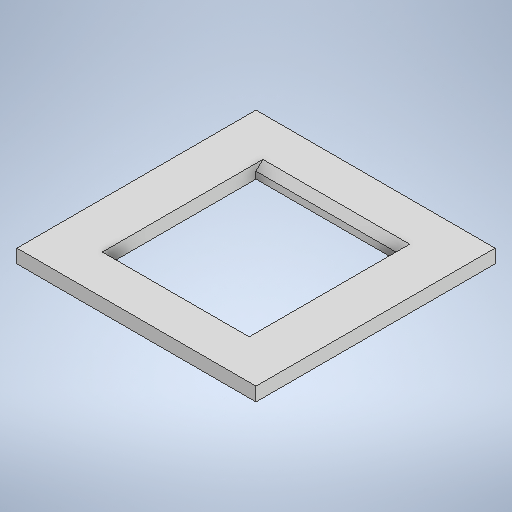
# Autodesk Inventor part: Plug_tester
Saved by Autodesk Inventor 2025 (Build 290162000, 162)
## iProperties
Created: 2024-12-15
Part Number: Plug_tester
Material: Generic
Document SubType Name: Modeling
Designer: ethan
Density: 1 g/cm^3
Appearance: Default
Author: ethan
Autodesk Inventor part; units mm, degrees
ref_plane "YZ Plane" through (0, 0, 0) normal (1, 0, 0) x (0, 1, 0)
ref_plane "XZ Plane" through (0, 0, 0) normal (0, 1, 0) x (-1, 0, 0)
ref_plane "XY Plane" through (0, 0, 0) normal (0, 0, 1) x (1, 0, 0)
sketch "Sketch1" plane through (0, 0, 0) normal (0, 1, 0) x (-1, 0, 0)
  line L0 (0, 0) -> (35, 0)
  line L1 (35, 0) -> (35, -35)
  line L2 (35, -35) -> (0, -35)
  line L3 (0, -35) -> (0, 0)
  line L4 (6.75, -6.75) -> (28.25, -6.75)
  line L5 (28.25, -6.75) -> (28.25, -28.25)
  line L6 (28.25, -28.25) -> (6.75, -28.25)
  line L7 (6.75, -28.25) -> (6.75, -6.75)
  line L8 (6.75, -6.75) -> (28.25, -28.25) construction
  line L9 (28.25, -6.75) -> (6.75, -28.25) construction
  point P0 (17.5, -17.5)
  dimension "d0" = 35
  dimension "d1" = 35
  dimension "d2" = 21.5
  dimension "d3" = 21.5
  constraints: 20 end point, 4 parallel, 2 horizontal, 2 midpoint, 2 perpendicular
  measures "d0" distance of L1.end L2.end
  measures "d1" distance of L0.end L1.end
  measures "d2" distance of L5.end L6.end
  measures "d3" distance of L4.end L5.end
extrude "Extrusion1" add sketch "Sketch1" along normal blind 2
chamfer "Chamfer1" distance 1 angle 45 2 edges at (-17.5, 2, -6.75) (-17.5, 2, -28.25)
body "Solid1"
